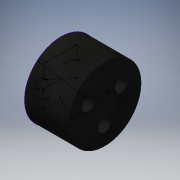
# Autodesk Inventor part: каркас
Saved by Autodesk Inventor 2019 (Build 230136000, 136)
## iProperties
Created: 2019-07-16
Part Number: каркас
Material: Пластмасса, непрозрачная, черная
Document SubType Name: Modeling
Designer: Boss
Mass: 0.429194 g
Surface Area: 3.95715 cm^2
Volume: 0.450834 cm^3
Density: 0.952 g/cm^3
Appearance: Гладкая — черная
Author: Boss
Autodesk Inventor part; units mm, degrees
ref_plane "YZ Plane" through (0, 0, 0) normal (1, 0, 0) x (0, 1, 0)
ref_plane "XZ Plane" through (0, 0, 0) normal (0, 1, 0) x (-1, 0, 0)
ref_plane "XY Plane" through (0, 0, 0) normal (0, 0, 1) x (1, 0, 0)
sketch "Эскиз1" plane through (0, 0, 0) normal (1, 0, 0) x (0, 1, 0)
  circle A0 centre (0, 0) radius 5
  circle A1 centre (0, -2.5) radius 0.6
  circle A2 centre (0, 0) radius 2.5 construction
  circle A3 centre (-2.2499, 1.09) radius 0.6
  circle A4 centre (2.2501, 1.0894) radius 0.6
  dimension "d1" = 10
  dimension "d2" = 2.5
  dimension "d3" = 1.2
  dimension "d24" = 5
  dimension "d25" = 1.2
  dimension "d26" = 1.2
  dimension "d27" = 4.5
  dimension "d29" = 1.09
  constraints: 5 centre point, 2 coincident, 2 point on circle, 1 vertical alignment
  measures "d1" diameter of A0
  measures "d2" distance of A1.centre point (0, 0)
  measures "d3" diameter of A1
  measures "d24" diameter of A2
  measures "d25" diameter of A3
  measures "d26" diameter of A4
  measures "d27" distance of A4.centre A3.centre
  measures "d29" vertical distance of point (0, 0) A3.centre
extrude "Выдавливание1" add sketch "Эскиз1" along normal blind 6 contours A0 | A3 | A4
hole "Отверстие2" at (6, 0, -2.5) direction (-1, 0, 0) diameter 1.7 depth 3
extrude "Выдавливание2" cut sketch "Эскиз1" along normal blind 6 contours A3 | A4
sketch "Эскиз2" plane through (6, 0, 0) normal (1, 0, 0) x (0, 0, -1)
  point P0 (0, 0)
  point P1 (-1.0881, 2.2526)
hole "Отверстие4" at (6, 2.2526, 1.0881) direction (-1, 0, 0) diameter 1.7 depth 3
sketch "Эскиз3" plane through (6, 0, 0) normal (1, 0, 0) x (0, 0, -1)
  point P0 (0, 0)
  point P1 (-1.0892, -2.2496)
hole "Отверстие5" at (6, -2.2496, 1.0892) direction (-1, 0, 0) diameter 1.7 depth 3
equation "\"d1\" = inside"
equation "\"d2\" = 0.5 * d0"
equation "\"d3\" = 2 * pin_small_rad"
equation "\"d17\" = pin_big_dia"
equation "\"inside\" = 10"
equation "\"pin_small_rad\" = 0.6"
equation "\"pin_big_dia\" = 1.7"
equation "\"d0\" = 5"
